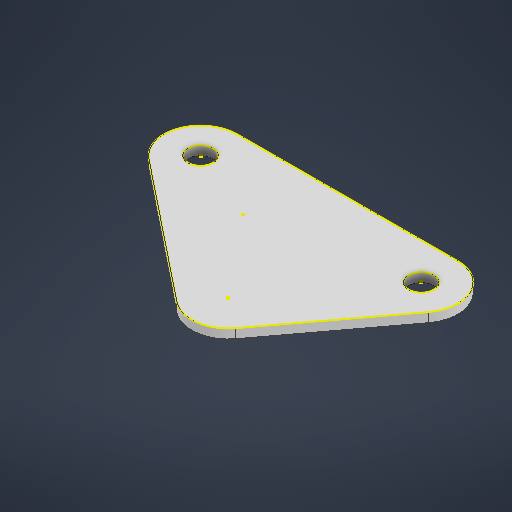
# Autodesk Inventor part: 1.25LadyBrown
Saved by Autodesk Inventor 2025 (Build 290162010, 162A)
## iProperties
Created: 2025-01-06
Part Number: 1.25LadyBrown
Material: Generic
Document SubType Name: Modeling
Designer: casey
Density: 1 g/cm^3
Appearance: Default
Mass: 1.89237 g
Surface Area: 26.677 cm^2
Volume: 1.89237 cm^3
Author: casey
Autodesk Inventor part; units mm, degrees
ref_plane "YZ Plane" through (0, 0, 0) normal (1, 0, 0) x (0, 1, 0)
ref_plane "XZ Plane" through (0, 0, 0) normal (0, 1, 0) x (-1, 0, 0)
ref_plane "XY Plane" through (0, 0, 0) normal (0, 0, 1) x (1, 0, 0)
sketch "Sketch1" plane through (0, 0, 0) normal (0, 1, 0) x (-1, 0, 0)
  circle A0 centre (-25.5886, -5.2973) radius 2.1844
  arc A1 (-30.2246, -0.9579) -> (-25.5886, -11.6473) centre (-25.5886, -5.2973) ccw
  circle A2 centre (12.5113, -5.2091) radius 2.1844
  arc A3 (12.526, -11.5591) -> (15.7227, 0.269) centre (12.5113, -5.2091) ccw
  line L0 (-25.5886, -11.6473) -> (12.526, -11.5591)
  arc A4 (12.526, -11.5591) -> (16.7749, -0.5033) centre (12.5113, -5.2091) ccw
  arc A5 (-30.8807, -1.7878) -> (-25.5886, -11.6473) centre (-25.5886, -5.2973) ccw
  line L1 (-11.315, -11.6142) -> (-11.315, 13.7858)
  circle A6 centre (-11.315, 13.7858) radius 6.35
  circle A7 centre (12.5113, -5.2091) radius 6.35
  circle A8 centre (-25.5886, -5.2973) radius 6.35
  line L2 (16.4697, -0.2438) -> (-7.3566, 18.751)
  line L3 (-16.4, 17.5892) -> (-30.6736, -1.4939)
  point P0 (0, 0)
  point P1 (-30.6736, -1.4939)
  dimension "d0" = 12.7
  dimension "d10" = 4.3688
  dimension "d11" = 12.7
  dimension "d16" = 38.1
  dimension "d19" = 25.4
  dimension "d20" = 12.7
  constraints: 10 point on circle, 8 end point, 7 centre point, 7 coincident, 3 tangent, 2 concentric, 1 point on line, 1 vertical, 10 other
  measures "d0" diameter of A1
  measures "d10" diameter of A2
  measures "d11" diameter of A3
  measures "d16" distance of A1.centre A2.centre
  measures "d19" distance of L1.start L1.end
  measures "d20" diameter of A6
extrude "Extrusion1" add sketch "Sketch1" along normal blind 1.5875
sketch "Sketch2" plane through (0, 1.5875, 0) normal (0, 1, 0) x (1, 0, 0)
  circle A0 centre (-25.1602, 5.259) radius 2.1844 projected
  circle A1 centre (25.5886, 5.2973) radius 2.1844 projected
  arc A2 (30.6736, 1.4939) -> (25.5886, 11.6473) centre (25.5886, 5.2973) ccw projected
  line L0 (25.5886, 11.609) -> (-25.1602, 11.609) projected
  line L1 (15.958, -14.3766) -> (30.2758, 0.9195) projected
  arc A3 (8.8667, -15.8933) -> (15.958, -14.3766) centre (11.3221, -10.0372) ccw projected
  line L2 (-27.6155, -0.5971) -> (8.8667, -15.8933) projected
  arc A4 (-25.1602, 11.609) -> (-27.6155, -0.5971) centre (-25.1602, 5.259) ccw projected
  point P0 (0, 0)
  point P1 (30.9319, 1.7495)
  dimension "d6" = 27.9962
sketch "Sketch3" plane through (0, 1.5875, 0) normal (0, 1, 0) x (1, 0, 0)
  line L0 (25.5886, 11.6473) -> (-12.526, 11.5591) projected
  arc A0 (-12.526, 11.5591) -> (-16.4697, 0.2438) centre (-12.5113, 5.2091) ccw projected
  line L1 (-16.4697, 0.2438) -> (7.3566, -18.751) projected
  arc A1 (7.3566, -18.751) -> (16.4, -17.5892) centre (11.315, -13.7858) ccw projected
  line L2 (16.4, -17.5892) -> (30.6736, 1.4939) projected
  arc A2 (30.6736, 1.4939) -> (25.5886, 11.6473) centre (25.5886, 5.2973) ccw projected
  circle A3 centre (25.5886, 5.2973) radius 2.1844 projected
  circle A4 centre (-12.5113, 5.2091) radius 2.1844 projected
  point P0 (0, 0)
body "Solid1"
